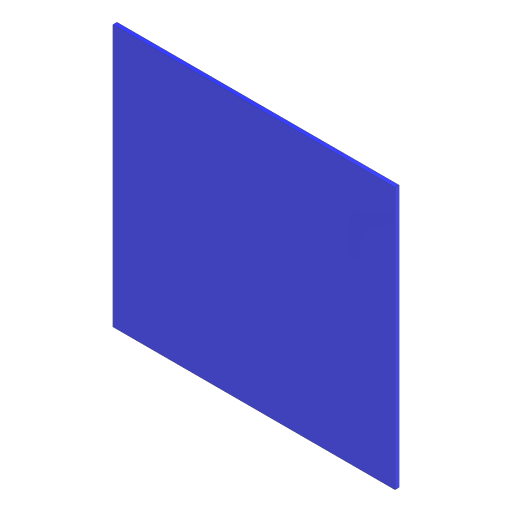
# Autodesk Inventor part: Передняя_Задняя фанера
Saved by Autodesk Inventor 2023.2 (Build 272271030, 271C)
## iProperties
Created: 2025-04-24
Part Number: Передняя_Задняя фанера
Material: Типовые
Document SubType Name: Modeling
Designer: Коноваленко
Density: 1 g/cm^3
Appearance: По умолчанию
Author: Коноваленко
Autodesk Inventor part; units mm, degrees
ref_plane "YZ Plane" through (0, 0, 0) normal (1, 0, 0) x (0, 1, 0)
ref_plane "XZ Plane" through (0, 0, 0) normal (0, 1, 0) x (-1, 0, 0)
ref_plane "XY Plane" through (0, 0, 0) normal (0, 0, 1) x (1, 0, 0)
sketch "Эскиз1" plane through (0, 0, 0) normal (0, 0, 1) x (1, 0, 0)
  line L0 (-140, -130) -> (140, -130)
  line L1 (140, -130) -> (140, 130)
  line L2 (140, 130) -> (-140, 130)
  line L3 (-140, 130) -> (-140, -130)
  line L4 (-140, -130) -> (140, 130) construction
  line L5 (140, -130) -> (-140, 130) construction
  point P0 (0, 0)
  dimension "d0" = 260
  dimension "d1" = 280
  constraints: 12 end point, 2 midpoint, 2 parallel, 1 horizontal, 1 perpendicular
  measures "d0" distance of L2.end L0.start
  measures "d1" distance of L0.start L0.end
extrude "Выдавливание1" add sketch "Эскиз1" along normal mid plane 4
